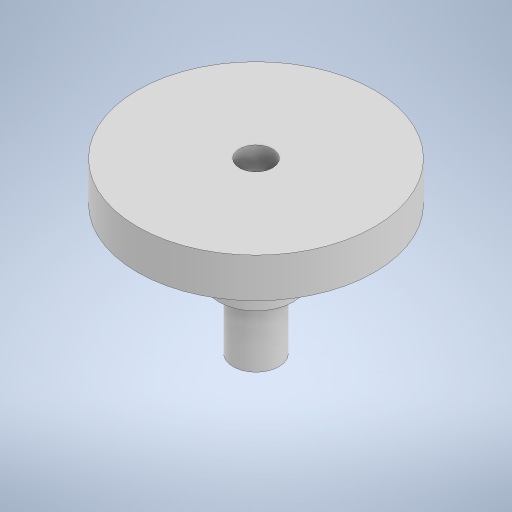
# Autodesk Inventor part: HOLE_CENTERINGRIG
Saved by Autodesk Inventor 2023 (Build 270158000, 158)
## iProperties
Created: 2022-07-31
Part Number: HOLE_CENTERINGRIG
Material: Generic
Document SubType Name: Modeling
Designer: plebbb
Density: 1 g/cm^3
Appearance: Default
Author: plebbb
Autodesk Inventor part; units mm, degrees
ref_plane "YZ Plane" through (0, 0, 0) normal (1, 0, 0) x (0, 1, 0)
ref_plane "XZ Plane" through (0, 0, 0) normal (0, 1, 0) x (-1, 0, 0)
ref_plane "XY Plane" through (0, 0, 0) normal (0, 0, 1) x (1, 0, 0)
sketch "Sketch1" plane through (0, 0, 0) normal (0, 0, 1) x (1, 0, 0)
  line L0 (2.1, 0) -> (2.1, 21.4)
  line L1 (2.1, 21.4) -> (4.7, 21.4)
  line L2 (4.7, 8) -> (2.9, 8)
  line L3 (2.9, 8) -> (2.9, 0)
  line L4 (2.9, 0) -> (2.1, 0)
  line L5 (4.7, 16.4) -> (15, 16.4)
  line L6 (15, 16.4) -> (15, 21.4)
  line L7 (15, 21.4) -> (4.7, 21.4)
  line L8 (4.7, 16.4) -> (4.7, 8)
  line L9 (0, 0) -> (0, 21.4) construction
  point P0 (2.5, 0)
  dimension "d0" = 2.1
  dimension "d1" = 4.7
  dimension "d3" = 8
  dimension "d4" = 2.9
  dimension "d5" = 5
  dimension "d6" = 16.4
  dimension "d7" = 15
  constraints: 20 end point, 6 perpendicular, 3 vertical, 1 horizontal, 1 horizontal alignment, 1 midpoint, 1 vertical alignment
  measures "d0" distance of L9.start L0.start
  measures "d1" horizontal distance of L1.end L9.start
  measures "d3" vertical distance of L2.start L3.end
  measures "d4" distance from line of L9.start L3
  measures "d5" distance of L5.end L6.end
  measures "d6" distance from line of L0.start L5
  measures "d7" horizontal distance of L9.start L6.end
revolve "Revolution1" add sketch "Sketch1" angle 360 about axis through (0, 0, 0) along (0, 1, 0)
body "Solid1"
